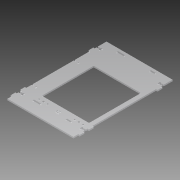
# Autodesk Inventor part: plastic_part_02
Saved by Autodesk Inventor 2013 (Build 170138000, 138)
## iProperties
Shininess: 20.0
Created: 2013-02-12
Part Number: plastic_part_02
Document SubType Name: Modeling
Designer: Noa Izumi
Material: Default
Density: 1 g/cm^3
Density: 0.0
Volumn: 0.0
Area: 0.0
PropertySet Name: Model Information
Control State: 0
Master: False
Checked Out: False
Author: Noa Izumi
Autodesk Inventor part; units mm, degrees
ref_plane "YZ Plane" through (0, 0, 0) normal (1, 0, 0) x (0, 1, 0)
ref_plane "XZ Plane" through (0, 0, 0) normal (0, 1, 0) x (-1, 0, 0)
ref_plane "XY Plane" through (0, 0, 0) normal (0, 0, 1) x (1, 0, 0)
sketch "Sketch1" plane through (0, 0, 0) normal (0, 0, 1) x (1, 0, 0)
  line L0 (0, 0) -> (140, 0)
  line L1 (140, 0) -> (140, 210)
  line L2 (140, 210) -> (0, 210)
  line L3 (0, 210) -> (0, 0)
  line L4 (-3, 10) -> (143, 10)
  line L5 (143, 10) -> (143, 20)
  line L6 (143, 20) -> (-3, 20)
  line L7 (-3, 20) -> (-3, 10)
  line L8 (-3, 30) -> (143, 30)
  line L9 (143, 30) -> (143, 40)
  line L10 (143, 40) -> (-3, 40)
  line L11 (-3, 40) -> (-3, 30)
  line L12 (-3, 185) -> (143, 185)
  line L13 (143, 185) -> (143, 175)
  line L14 (143, 175) -> (-3, 175)
  line L15 (-3, 175) -> (-3, 185)
  dimension "d0" = 140
  dimension "d1" = 210
  dimension "d14" = 146
  dimension "d15" = 10
  dimension "d16" = 3
  dimension "d17" = 10
  dimension "d18" = 10
  dimension "d19" = 10
  dimension "d23" = 10
  dimension "d60" = 146
  dimension "d191" = 3
  dimension "d192" = 25
  constraints: 32 end point, 8 parallel, 4 horizontal, 4 perpendicular, 1 point on line
  measures "d0" distance of L0.start L0.end
  measures "d1" distance of L2.end L0.start
  measures "d14" distance of L4.start L4.end
  measures "d15" distance of L6.end L4.start
  measures "d16" distance between parallel lines of L3 L7
  measures "d17" distance between parallel lines of L0 L4
  measures "d18" distance of L10.end L8.start
  measures "d19" distance between parallel lines of L6 L8
  measures "d23" distance of L14.end L12.start
  measures "d60" distance of L13.end L14.end
  measures "d191" distance between parallel lines of L3 L15
  measures "d192" distance between parallel lines of L2 L12
extrude "Extrusion1" add sketch "Sketch1" along normal blind 3
sketch "Sketch2" plane through (0, 0, 3) normal (0, 0, 1) x (1, 0, 0)
  line L0 (140, 30) -> (140, 20) projected
  line L1 (143, 30) -> (140, 30) projected
  line L2 (140, 190) -> (140, 185) projected
  line L3 (0, 185) -> (0, 190) projected
  line L4 (0, 30) -> (-3, 30) projected
  line L5 (0, 20) -> (0, 30) projected
  line L6 (0, 191.5) -> (9, 191.5)
  line L7 (9, 191.5) -> (9, 188.5)
  line L8 (9, 188.5) -> (0, 188.5)
  line L9 (0, 188.5) -> (0, 191.5)
  line L10 (9, 192.75) -> (6.7, 192.75)
  line L11 (6.7, 192.75) -> (6.7, 187.25)
  line L12 (6.7, 187.25) -> (9, 187.25)
  line L13 (9, 187.25) -> (9, 192.75)
  line L14 (140, 191.5) -> (131, 191.5)
  line L15 (131, 191.5) -> (131, 188.5)
  line L16 (131, 188.5) -> (140, 188.5)
  line L17 (140, 188.5) -> (140, 191.5)
  line L18 (131, 192.75) -> (133.3, 192.75)
  line L19 (133.3, 192.75) -> (133.3, 187.25)
  line L20 (133.3, 187.25) -> (131, 187.25)
  line L21 (131, 187.25) -> (131, 192.75)
  line L22 (0, 26.5) -> (9, 26.5)
  line L23 (9, 26.5) -> (9, 23.5)
  line L24 (9, 23.5) -> (0, 23.5)
  line L25 (0, 23.5) -> (0, 26.5)
  line L26 (9, 27.75) -> (6.7, 27.75)
  line L27 (6.7, 27.75) -> (6.7, 22.25)
  line L28 (6.7, 22.25) -> (9, 22.25)
  line L29 (9, 22.25) -> (9, 27.75)
  line L30 (140, 26.5) -> (131, 26.5)
  line L31 (131, 26.5) -> (131, 23.5)
  line L32 (131, 23.5) -> (140, 23.5)
  line L33 (140, 23.5) -> (140, 26.5)
  line L34 (131, 27.75) -> (133.3, 27.75)
  line L35 (133.3, 27.75) -> (133.3, 22.25)
  line L36 (133.3, 22.25) -> (131, 22.25)
  line L37 (131, 22.25) -> (131, 27.75)
  line L38 (0, 210) -> (140, 210) projected
  dimension "d26" = 3
  dimension "d29" = 2.3
  dimension "d30" = 0
  dimension "d31" = 5.5
  dimension "d33" = 3
  dimension "d34" = 9
  dimension "d35" = 5.5
  dimension "d36" = 2.3
  dimension "d38" = 9
  dimension "d39" = 3
  dimension "d40" = 3.5
  dimension "d41" = 2.3
  dimension "d42" = 5.5
  dimension "d43" = 2.25
  dimension "d44" = 9
  dimension "d45" = 2.3
  dimension "d46" = 2.25
  dimension "d47" = 5.5
  dimension "d188" = 18.5
  dimension "d189" = 1.25
  dimension "d190" = 1.25
  constraints: 64 end point, 16 parallel, 8 horizontal, 8 perpendicular, 5 point on line
  measures "d26" distance of L8.end L6.start
  measures "d29" distance of L10.start L10.end
  measures "d30" distance between parallel lines of L7 L13
  measures "d31" distance of L12.end L10.start
  measures "d33" distance of L14.end L15.end
  measures "d34" distance of L15.end L16.end
  measures "d35" distance of L20.end L18.start
  measures "d36" distance of L18.start L18.end
  measures "d38" distance of L22.start L22.end
  measures "d39" distance of L22.end L23.end
  measures "d40" distance between parallel lines of L22 L4
  measures "d41" distance of L27.end L28.end
  measures "d42" distance of L28.end L26.start
  measures "d43" distance between parallel lines of L4 L26
  measures "d44" distance of L30.start L30.end
  measures "d45" distance of L34.start L34.end
  measures "d46" distance between parallel lines of L1 L34
  measures "d47" distance of L36.end L34.start
  measures "d188" distance between parallel lines of L38 L6
  measures "d189" distance between parallel lines of L6 L10
  measures "d190" distance between parallel lines of L14 L18
extrude "Extrusion2" cut sketch "Sketch2" against normal through all
sketch "Sketch3" plane through (0, 0, 3) normal (0, 0, 1) x (1, 0, 0)
  line L0 (0, 0) -> (0, 10) projected
  line L1 (140, 0) -> (0, 0) projected
  line L2 (140, 10) -> (140, 0) projected
  line L3 (30, 23.5) -> (45, 23.5)
  line L4 (45, 23.5) -> (45, 26.5)
  line L5 (45, 26.5) -> (30, 26.5)
  line L6 (30, 26.5) -> (30, 23.5)
  line L7 (100, 23.5) -> (110, 23.5)
  line L8 (110, 23.5) -> (110, 26.5)
  line L9 (110, 26.5) -> (100, 26.5)
  line L10 (100, 26.5) -> (100, 23.5)
  line L11 (0, 210) -> (140, 210) projected
  line L12 (30, 204.5) -> (45, 204.5)
  line L13 (45, 204.5) -> (45, 201.5)
  line L14 (45, 201.5) -> (30, 201.5)
  line L15 (30, 201.5) -> (30, 204.5)
  line L16 (100, 204.5) -> (110, 204.5)
  line L17 (110, 204.5) -> (110, 201.5)
  line L18 (110, 201.5) -> (100, 201.5)
  line L19 (100, 201.5) -> (100, 204.5)
  line L20 (140, 210) -> (140, 200) projected
  line L21 (0, 200) -> (0, 210) projected
  dimension "d50" = 15
  dimension "d51" = 3
  dimension "d52" = 23.5
  dimension "d53" = 10
  dimension "d54" = 3
  dimension "d55" = 23.5
  dimension "d56" = 30
  dimension "d57" = 30
  dimension "d91" = 15
  dimension "d92" = 3
  dimension "d93" = 5.5
  dimension "d134" = 30
  dimension "d135" = 30
  dimension "d136" = 10
  dimension "d148" = 5.5
  dimension "d149" = 3
  constraints: 32 end point, 8 parallel, 4 horizontal, 4 perpendicular
  measures "d50" distance of L3.start L3.end
  measures "d51" distance of L3.end L4.end
  measures "d52" distance between parallel lines of L1 L3
  measures "d53" distance of L7.start L7.end
  measures "d54" distance of L7.end L8.end
  measures "d55" distance between parallel lines of L1 L7
  measures "d56" distance between parallel lines of L6 L0
  measures "d57" distance between parallel lines of L2 L8
  measures "d91" distance of L12.start L12.end
  measures "d92" distance of L14.end L12.start
  measures "d93" distance between parallel lines of L12 L11
  measures "d134" distance between parallel lines of L15 L21
  measures "d135" distance between parallel lines of L20 L17
  measures "d136" distance of L16.start L16.end
  measures "d148" distance between parallel lines of L16 L11
  measures "d149" distance of L18.end L16.start
extrude "Extrusion3" cut sketch "Sketch3" against normal through all
sketch "Sketch7" plane through (0, 0, 3) normal (0, 0, 1) x (1, 0, 0)
  line L0 (30, 26.5) -> (45, 26.5) projected
  line L1 (140, 175) -> (140, 40) projected
  line L2 (100, 26.5) -> (110, 26.5) projected
  point P0 (43.5, 33)
  point P1 (118.5, 33)
  dimension "d94" = 6.5
  dimension "d95" = 75
  dimension "d96" = 21.5
  dimension "d115" = 6.5
  measures "d94" distance from line of L0 point (43.5, 33)
  measures "d95" distance of point (118.5, 33) point (43.5, 33)
  measures "d96" distance from line of L1 point (118.5, 33)
  measures "d115" distance from line of L2 point (118.5, 33)
hole "Hole3" at (43.5, 33, 3) at (118.5, 33, 3) direction (0, 0, -1) diameter 4 end through all
sketch "Sketch8" plane through (0, 0, 3) normal (0, 0, 1) x (1, 0, 0)
  circle A0 centre (43.5, 33) radius 2 projected
  circle A1 centre (118.5, 33) radius 2 projected
  point P0 (34.5, 33)
  point P1 (52.5, 33)
  point P2 (109.5, 33)
  point P3 (127.5, 33)
  dimension "d104" = 9
  dimension "d105" = 9
  dimension "d106" = 9
  dimension "d107" = 9
  dimension "d116" = 0
  dimension "d117" = 0
  dimension "d145" = 0
  dimension "d146" = 0
  measures "d104" distance of A0.centre point (34.5, 33)
  measures "d105" distance of point (52.5, 33) A0.centre
  measures "d106" distance of A1.centre point (109.5, 33)
  measures "d107" distance of point (127.5, 33) A1.centre
  measures "d116" vertical distance of A0.centre point (34.5, 33)
  measures "d117" vertical distance of A1.centre point (109.5, 33)
  measures "d145" vertical distance of A0.centre point (52.5, 33)
  measures "d146" vertical distance of A1.centre point (127.5, 33)
hole "Hole4" at (34.5, 33, 3) at (52.5, 33, 3) at (109.5, 33, 3) at (127.5, 33, 3) direction (0, 0, -1) diameter 3 end through all
sketch "Sketch9" plane through (0, 0, 3) normal (0, 0, 1) x (1, 0, 0)
  circle A0 centre (43.5, 33) radius 2 projected
  circle A1 centre (118.5, 33) radius 2 projected
  line L0 (31, 42) -> (131, 42)
  line L1 (131, 42) -> (131, 152)
  line L2 (131, 152) -> (31, 152)
  line L3 (31, 152) -> (31, 42)
  dimension "d118" = 100
  dimension "d119" = 110
  dimension "d120" = 9
  dimension "d121" = 12.5
  constraints: 8 end point, 2 parallel, 1 horizontal, 1 perpendicular
  measures "d118" distance of L0.start L0.end
  measures "d119" distance of L2.end L0.start
  measures "d120" distance from line of A0.centre L0
  measures "d121" distance from line of A1.centre L1
extrude "Extrusion4" cut sketch "Sketch9" against normal through all contours L3 L2 L1 L0
fillet "Fillet1" radius 2 4 edges at (31, 152, 1.5) (31, 42, 1.5) (131, 42, 1.5) (131, 152, 1.5)
sketch "Sketch14" plane through (0, 0, 3) normal (0, 0, 1) x (1, 0, 0)
  line L0 (74.5, 32) -> (76, 32)
  line L1 (76, 32) -> (76, 28)
  line L2 (76, 28) -> (74.5, 28)
  line L3 (74.5, 28) -> (74.5, 32)
  line L4 (140, 175) -> (140, 40) projected
  line L5 (140, 0) -> (0, 0) projected
  line L6 (77.75, 32) -> (80.25, 32)
  line L7 (80.25, 32) -> (80.25, 33.4)
  line L8 (80.25, 33.4) -> (77.75, 33.4)
  line L9 (77.75, 33.4) -> (77.75, 32)
  line L10 (77.75, 28) -> (80.25, 28)
  line L11 (80.25, 28) -> (80.25, 26.6)
  line L12 (80.25, 26.6) -> (77.75, 26.6)
  line L13 (77.75, 26.6) -> (77.75, 28)
  dimension "d159" = 1.5
  dimension "d160" = 4
  dimension "d165" = 28
  dimension "d166" = 64
  dimension "d167" = 2.5
  dimension "d168" = 1.4
  dimension "d171" = 1.4
  dimension "d193" = 0
  dimension "d194" = 0
  constraints: 24 end point, 6 parallel, 3 horizontal, 3 perpendicular
  measures "d159" distance of L0.start L0.end
  measures "d160" distance of L0.end L1.end
  measures "d165" distance between parallel lines of L5 L2
  measures "d166" distance between parallel lines of L4 L1
  measures "d167" distance of L7.end L8.end
  measures "d168" distance of L6.end L7.end
  measures "d171" distance of L10.end L11.end
  measures "d193" distance between parallel lines of L0 L6
  measures "d194" distance between parallel lines of L2 L10
extrude "Extrusion5" cut sketch "Sketch14" against normal through all
sketch "草圖15" plane through (0, 0, 3) normal (0, 0, 1) x (1, 0, 0)
  line L0 (33, 152) -> (129, 152) projected
  line L1 (0, 40) -> (0, 175) projected
  line L2 (-3, 40) -> (0, 40) projected
  line L3 (0, 50.75) -> (1.6, 50.75)
  line L4 (1.6, 50.75) -> (1.6, 53.25)
  line L5 (1.6, 53.25) -> (0, 53.25)
  line L6 (0, 53.25) -> (0, 50.75)
  line L7 (7.775, 53.25) -> (9.175, 53.25)
  line L8 (9.175, 53.25) -> (9.175, 50.75)
  line L9 (9.175, 50.75) -> (7.775, 50.75)
  line L10 (7.775, 50.75) -> (7.775, 53.25)
  line L11 (0, 143.25) -> (1.6, 143.25)
  line L12 (1.6, 143.25) -> (1.6, 140.75)
  line L13 (1.6, 140.75) -> (0, 140.75)
  line L14 (0, 140.75) -> (0, 143.25)
  line L15 (7.775, 143.25) -> (9.175, 143.25)
  line L16 (9.175, 143.25) -> (9.175, 140.75)
  line L17 (9.175, 140.75) -> (7.775, 140.75)
  line L18 (7.775, 140.75) -> (7.775, 143.25)
  dimension "d173" = 2.5
  dimension "d175" = 1.6
  dimension "d176" = 10.75
  dimension "d177" = 1.4
  dimension "d178" = 6.175
  dimension "d179" = 2.5
  dimension "d180" = 8.75
  dimension "d181" = 1.4
  dimension "d182" = 6.175
  constraints: 32 end point, 8 parallel, 4 horizontal, 4 perpendicular, 3 point on line
  measures "d173" distance of L3.end L4.end
  measures "d175" distance of L4.end L5.end
  measures "d176" distance between parallel lines of L2 L3
  measures "d177" distance of L7.start L7.end
  measures "d178" distance between parallel lines of L10 L4
  measures "d179" distance of L11.end L12.end
  measures "d180" distance between parallel lines of L0 L11
  measures "d181" distance of L15.start L15.end
  measures "d182" distance between parallel lines of L18 L12
extrude "擠出6" cut sketch "草圖15" against normal through all
